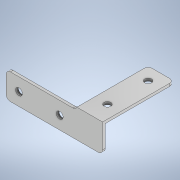
# Autodesk Inventor part: TH22_CP_fitting_R_sn
Saved by Autodesk Inventor 2022 (Build 260153070, 153G)
## iProperties
Created: 2021-12-08
Part Number: TH22_CP_fitting_R_sn
Material: アルミニウム 6061-AHC
Document SubType Name: Modeling
Designer: 中島 青蔵
Density: 2.7 g/cm^3
Appearance: アルミニウム - ダーク
Author: 中島 青蔵
Autodesk Inventor part; units mm, degrees
ref_plane "YZ Plane" through (0, 0, 0) normal (1, 0, 0) x (0, 1, 0)
ref_plane "XZ Plane" through (0, 0, 0) normal (0, 1, 0) x (-1, 0, 0)
ref_plane "XY Plane" through (0, 0, 0) normal (0, 0, 1) x (1, 0, 0)
sketch "スケッチ1" plane through (0, 0, 0) normal (0, 0, 1) x (1, 0, 0)
  line L0 (0, 0) -> (45, 0)
  line L1 (45, 0) -> (45, 12)
  line L2 (45, 12) -> (0, 12)
  line L3 (0, 12) -> (0, 0)
  dimension "d0" = 45
  dimension "d1" = 12
  constraints: 8 end point
  measures "d0" distance of L2.end L1.end
  measures "d1" distance of L1.end L0.end
extrude "押し出し1" add sketch "スケッチ1" along normal blind 1.25
sketch "スケッチ2" plane through (0, 0, 1.25) normal (0, 0, 1) x (1, 0, 0)
  line L0 (45, 12) -> (0, 12) projected
  line L1 (45, 12) -> (33, 12)
  line L2 (33, 12) -> (33, 13.25)
  line L3 (33, 13.25) -> (45, 13.25)
  line L4 (45, 13.25) -> (45, 12)
  point P0 (0, 0)
  dimension "d4" = 12
  dimension "d5" = 1.25
  constraints: 8 end point
  measures "d4" distance of L2.end L3.end
  measures "d5" distance of L1.end L2.end
extrude "押し出し2" add sketch "スケッチ2" against normal blind 33.25
sketch "スケッチ3" plane through (0, 0, 0) normal (0, 0, -1) x (-1, 0, 0)
  line L0 (-45, 0) -> (-45, 12) projected
  point P0 (0, 0)
  point P1 (-6, 6)
  point P2 (-25, 6)
  dimension "d8" = 20
  dimension "d9" = 39
  measures "d8" distance from line of L0 point (-25, 6)
  measures "d9" distance from line of L0 point (-6, 6)
hole "穴1" at (6, 6, 0) at (25, 6, 0) direction (0, 0, 1) diameter 3.2 end through all
sketch "スケッチ4" plane through (33, 12, 0) normal (0, -1, 0) x (1, 0, 0)
  line L0 (-33, 0) -> (12, 0) projected
  point P0 (6, -26)
  point P1 (6, -7)
  dimension "d17" = 7
  dimension "d18" = 26
  measures "d17" distance from line of L0 point (6, -7)
  measures "d18" distance from line of L0 point (6, -26)
hole "穴2" at (39, 12, -26) at (39, 12, -7) direction (0, 1, 0) diameter 3.2 end through all
fillet "フィレット1" radius 2 6 edges at (33, 12.625, -32) (45, 12.625, -32) (45, 0, 0.625) (0, 0, 0.625) (0, 12, 0.625) (33, 12, 0.625)
